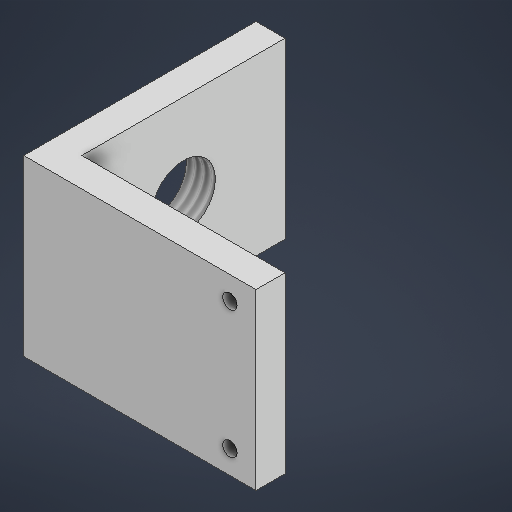
# Autodesk Inventor part: Soporte
Saved by Autodesk Inventor 2026.3 (Build 303398000, 398)
## iProperties
Created: 2026-06-14
Part Number: Soporte
Material: Genérico
Document SubType Name: Modeling
Designer: ASUS
Density: 1 g/cm^3
Appearance: Valor por defecto
Author: ASUS
Autodesk Inventor part; units mm, degrees
ref_plane "YZ Plane" through (0, 0, 0) normal (1, 0, 0) x (0, 1, 0)
ref_plane "XZ Plane" through (0, 0, 0) normal (0, 1, 0) x (-1, 0, 0)
ref_plane "Plano de trabajo1" through (0, -46.2161, 0) normal (0, 0, 1) x (-1, 0, 0)
sketch "Boceto1" plane through (0, -46.2161, 0) normal (0, 0, 1) x (-1, 0, 0)
  line L0 (14.8515, 14.9812) -> (54.8515, 14.9812)
  line L1 (14.8515, -15) -> (14.8515, 14.9812)
  line L2 (54.8515, -15) -> (14.8515, -15)
  line L3 (54.8515, 14.9812) -> (54.8515, -15)
  circle A0 centre (19.3515, 11) radius 1.25
  circle A1 centre (19.3515, -11.0188) radius 1.25
  point P0 (0, -46.2161)
  constraints: 8 end point, 2 centre point, 2 horizontal, 2 vertical, 8 other
extrude "Extrusión1" add sketch "Boceto1" against normal blind 5
sketch "Boceto2" plane through (0, -46.2161, -5) normal (0, 0, -1) x (-1, 0, 0)
  line L0 (54.8515, -14.9812) -> (54.8515, 15) projected
  line L1 (54.8515, 15) -> (14.8515, 15) projected
  line L2 (54.8515, -14.9812) -> (49.8515, -14.9812)
  line L3 (49.8515, -14.9812) -> (49.8515, 15)
  line L4 (49.8515, 15) -> (54.8515, 15)
  line L5 (54.8515, 15) -> (54.8515, -14.9812)
  point P0 (0, 46.2161)
  dimension "d2" = 5
  constraints: 8 end point, 2 parallel, 1 horizontal, 1 perpendicular, 1 point on line
  measures "d2" distance of L3.end L4.end
extrude "Extrusión2" add sketch "Boceto2" along normal blind 35
sketch "Boceto3" plane through (-49.8515, -61.1974, -5) normal (1, 0, 0) x (0, 0, -1)
  line L0 (0, 0) -> (35, 0)
  line L1 (35, 0) -> (35, 29.9812)
  line L2 (35, 29.9812) -> (0, 29.9812)
  line L3 (0, 29.9812) -> (0, 0)
  line L4 (0, 0) -> (35, 0) projected
  line L5 (0, 29.9812) -> (35, 29.9812) projected
  circle A0 centre (17.5, 14.9906) radius 5.5
  point P0 (-5, 61.1974)
  dimension "d5" = 11
  constraints: 8 end point, 2 parallel, 1 centre point, 1 horizontal, 1 perpendicular
  measures "d5" diameter of A0
extrude "Extrusión3" cut sketch "Boceto3" against normal blind 35 contours A0
thread "Rosca1" size "M11x1.5" class "6H" standard "ANSI Metric M Profile" full length
